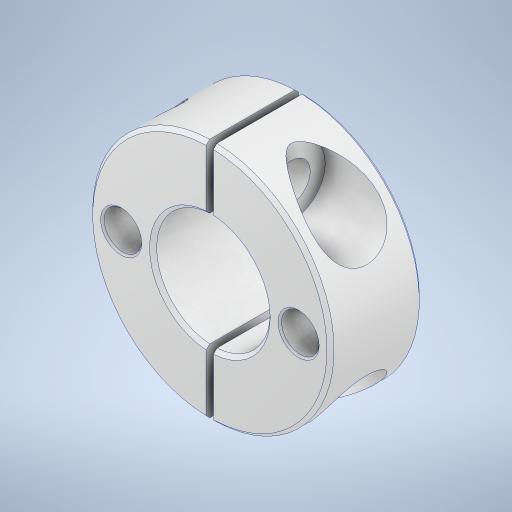
# Autodesk Inventor part: Shaft Clamp
Saved by Autodesk Inventor 2024 (Build 280153000, 153)
## iProperties
Created: 2024-12-28
Part Number: Shaft Clamp
Material: Aluminum 6061
Document SubType Name: Modeling
Designer: Ishaan
Density: 2.7 g/cm^3
Appearance: Aluminum - Flat
Author: Ishaan
Autodesk Inventor part; units mm, degrees
ref_plane "XZ Plane" through (0, 0, 0) normal (0, 1, 0) x (-1, 0, 0)
sketch "Sketch1" plane through (0, 0, 0) normal (0, 0, 1) x (1, 0, 0)
  circle A0 centre (0, 0) radius 8
  circle A1 centre (0, 0) radius 17
  line L0 (0.5, -17) -> (-0.5, -17)
  line L1 (-0.5, -17) -> (-0.5, 17)
  line L2 (-0.5, 17) -> (0.5, 17)
  line L3 (0.5, 17) -> (0.5, -17)
  line L4 (0.5, -17) -> (-0.5, 17) construction
  line L5 (-0.5, -17) -> (0.5, 17) construction
  point P0 (0.5, -7.9844)
  point P1 (0.5, -16.9926)
  point P2 (0.5, 16.9926)
  point P3 (0.5, 7.9844)
  point P4 (-0.5, 7.9844)
  point P5 (-0.5, 16.9926)
  point P6 (-0.5, -16.9926)
  point P7 (-0.5, -7.9844)
  dimension "d0" = 16
  dimension "d1" = 34
  dimension "d2" = 1
  constraints: 12 end point, 2 centre point, 2 coincident, 2 midpoint, 2 parallel, 1 horizontal, 1 perpendicular, 1 tangent
  measures "d0" diameter of A0
  measures "d1" diameter of A1
  measures "d2" distance of L1.end L2.end
extrude "Extrusion1" add sketch "Sketch1" along normal mid plane 13 contours A0 L3 A1 | A0 L1 A1
chamfer "Chamfer1" distance 0.5 angle 45 8 edges at (-8, 0, 6.5) (8, 0, 6.5) (17, 0, 6.5) (-17, 0, 6.5) (-17, 0, -6.5) (17, 0, -6.5) (-8, 0, -6.5) (8, 0, -6.5)
ref_plane "Work Plane1" through (17, 0, 0) normal (1, 0, 0) x (0, 1, 0)
sketch "Sketch2" plane through (17, 0, 0) normal (1, 0, 0) x (0, 1, 0)
  line L0 (16.4924, -6.5) -> (8.4853, -6.5) construction
  line L1 (16.9926, -6) -> (16.4924, -6.5) construction
  line L2 (16.9926, 6) -> (16.9926, -6) construction
  line L3 (16.4924, 6.5) -> (16.9926, 6) construction
  line L4 (8.4853, 6.5) -> (16.4924, 6.5) construction
  line L5 (7.9844, -6) -> (7.9844, 6) construction
  line L6 (-7.9844, -6) -> (-7.9844, 6) construction
  line L7 (-16.4924, 6.5) -> (-8.4853, 6.5) construction
  line L8 (-16.9926, 6) -> (-16.4924, 6.5) construction
  line L9 (-16.9926, -6) -> (-16.9926, 6) construction
  line L10 (-16.4924, -6.5) -> (-16.9926, -6) construction
  line L11 (-8.4853, -6.5) -> (-16.4924, -6.5) construction
  line L12 (-11.5, 0) -> (11.5, 0) construction
  point P0 (0, 0)
  point P1 (0, 0)
  dimension "d8" = 23
  constraints: 2 end point, 1 coincident, 1 horizontal, 1 midpoint, 4 other
  measures "d8" distance of L12.start L12.end
ref_plane "Work Plane2" through (5, 0, 0) normal (1, 0, 0) x (0, 1, 0)
hole "Hole1" at (17, 11.5, 0) at (17, -11.5, 0) direction (-1, 0, 0) diameter 4.134 end through all counterbore diameter 9.5 counterbore depth 12 thread size "M5x0.8" class "6H" standard "ANSI Metric M Profile"
sketch "Sketch3" plane through (5, 11.5, 0) normal (1, 0, 0) x (0, 0, -1)
  arc A0 (-0.1352, 4.7481) -> (0.1352, 4.7481) centre (0, 0) ccw projected
  circle A1 centre (0, 0) radius 2.067 projected
  arc A2 (0.1352, -27.7481) -> (-0.1352, -27.7481) centre (0, -23) ccw projected
  circle A3 centre (0, -23) radius 2.067 projected
  line L0 (0.1352, -27.7481) -> (-0.1352, -27.7481) projected
  line L1 (-0.1352, 4.7481) -> (0.1352, 4.7481) projected
  point P0 (0, -11.5)
hole "Hole2" at (5, 11.5, 0) at (5, -11.5, 0) direction (-1, 0, 0) diameter 5.3 depth 4.5
sketch "Sketch4" plane through (0, 0, -6.5) normal (0, 0, -1) x (-1, 0, 0)
  line L0 (-12.5, 0) -> (12.5, 0) construction
  line L1 (0, 0) -> (8, -6) construction
  line L2 (8, -6) -> (12.5, 0) construction
  dimension "d24" = 10
  dimension "d26" = 25
  dimension "d27" = 7.5
  constraints: 6 end point, 2 coincident, 1 horizontal, 1 midpoint, 1 perpendicular
  measures "d24" distance of L1.start L1.end
  measures "d26" distance of L0.start L0.end
  measures "d27" distance of L1.end L0.end
hole "Hole3" at (12.5, 0, -6.5) at (-12.5, 0, -6.5) direction (0, 0, 1) diameter 5.3 end through all
chamfer "Chamfer2" distance 0.25 angle 45 4 edges at (-12.5, -2.65, 6.5) (12.5, -2.65, 6.5) (-12.5, -2.65, -6.5) (12.5, -2.65, -6.5)
body "Solid1"
